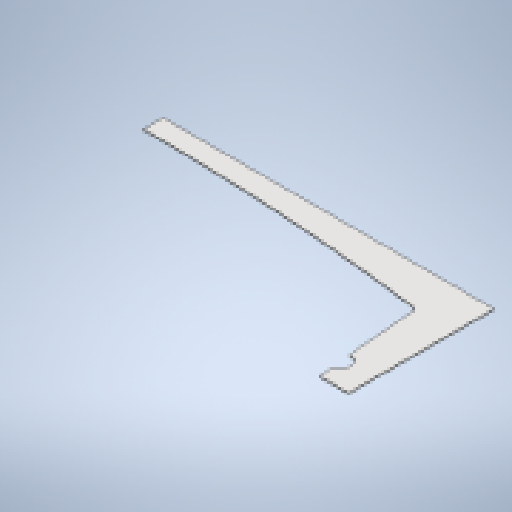
# Autodesk Inventor part: МОО 041 шпангоут спина 1
Saved by Autodesk Inventor 2024.2 (Build 282272000, 272)
## iProperties
Created: 2024-04-28
Part Number: МОО 041 шпангоут спина 1
Material: Generic
Document SubType Name: Sheet Metal
Designer: admin
Density: 1 g/cm^3
Sheet Metal Rule: Default_mm
Appearance: Default
Author: admin
Autodesk Inventor part; units mm, degrees
ref_plane "YZ Plane" through (0, 0, 0) normal (1, 0, 0) x (0, 1, 0)
ref_plane "XZ Plane" through (0, 0, 0) normal (0, 1, 0) x (-1, 0, 0)
ref_plane "XY Plane" through (0, 0, 0) normal (0, 0, 1) x (1, 0, 0)
sketch "Sketch1" plane through (0, 0, 0) normal (0, 0, 1) x (1, 0, 0)
  line L0 (-750, 0) -> (750, 0) construction
  line L1 (750, 0) -> (750, -2700) construction
  line L2 (750, -2700) -> (-750, -2700) construction
  line L3 (-750, -2700) -> (-750, 0) construction
  line L4 (800, 50) -> (-800, 50) construction
  line L5 (-800, 50) -> (-800, -2750) construction
  line L6 (-800, -2750) -> (800, -2750) construction
  line L7 (800, -2750) -> (800, 50) construction
  line L8 (-850, 100) -> (850, 100)
  line L9 (850, 100) -> (850, -2800) construction
  line L10 (850, -2800) -> (-850, -2800) construction
  line L11 (-850, -2800) -> (-850, 100) construction
  arc A0 (750, 0) -> (745.2706, 0.6314) centre (0, -5600) ccw construction
  line L12 (-750, -2100) -> (750, -2100) construction
  line L13 (114.1118, -2698.3696) -> (750, -2100) construction
  arc A1 (750, -2100) -> (770.156, -238.4205) centre (-10250, -1050) ccw construction
  line L14 (750, 0) -> (749.6018, -2.9735) construction
  arc A2 (750, -3.0268) -> (0, 47) centre (-0.2, -5603) ccw construction
  line L15 (750, 0) -> (747.0136, -0.2851) construction
  arc A3 (767.1641, -238.6409) -> (747.4657, -5.0326) centre (-10252.9895, -1050.2527) ccw construction
  arc A4 (750.4522, -4.7486) -> (745.2706, 0.6314) centre (744.4791, -5.3162) ccw
  arc A5 (747.4657, -5.0326) -> (744.8748, -2.3426) centre (744.4792, -5.3164) ccw construction
  line L16 (750, -2100) -> (752.9864, -2100.2851) construction
  arc A6 (752.9864, -2100.2851) -> (771.2831, -213.263) centre (-10246.9891, -1050.0292) ccw
  line L17 (750, -2100) -> (752.0559, -2102.1848) construction
  arc A7 (749.1768, -2100.7746) -> (750.1074, -2098.8746) centre (747.1209, -2098.5898) ccw construction
  line L18 (0, -2697) -> (110, -2697) construction
  line L19 (112.0559, -2696.1848) -> (690.4112, -2151.9536) construction
  arc A8 (110, -2700) -> (114.1118, -2698.3696) centre (110, -2694) ccw construction
  arc A9 (110, -2697) -> (112.0559, -2696.1848) centre (110, -2694) ccw construction
  line L20 (690.4112, -2151.9536) -> (692.4671, -2154.1384) construction
  line L21 (752.0559, -2102.1848) -> (676.3163, -2173.4556) construction
  line L22 (676.3163, -2173.4556) -> (674.2605, -2171.2708) construction
  arc A10 (747.4657, -5.0326) -> (747.0136, -0.2851) centre (-10252.9895, -1050.2527) ccw construction
  arc A11 (745.2706, 0.6314) -> (0, 50) centre (0, -5600) ccw
  arc A12 (750.4522, -4.7486) -> (750, 0) centre (-10250, -1050) ccw construction
  line L23 (770.156, -238.4205) -> (767.1641, -238.6409) construction
  line L24 (768.2917, -213.4901) -> (771.2831, -213.263) construction
  arc A13 (770.156, -238.4205) -> (750.4522, -4.7486) centre (-10250, -1050) ccw
  line L25 (0, 100) -> (0, 50)
  line L26 (0, -2700) -> (0, -2697) construction
  line L27 (0, 47) -> (0, 0) construction
  line L28 (0, 50) -> (0, 47) construction
  arc A14 (752.0559, -2102.1848) -> (752.9864, -2100.2851) centre (749.9998, -2099.9999) ccw construction
  circle A15 centre (768.2917, -213.4901) radius 25
  line L29 (850, -253.0064) -> (774.6194, -258.4205)
  arc A16 (800, 50) -> (0, 100) centre (0, -6325) ccw construction
  arc A17 (824.491, -254.8386) -> (800, 50) centre (-10587.7814, -1018.3062) ccw construction
  line L30 (824.491, -254.8386) -> (824.491, 100)
  point P0 (0, 0)
  point P1 (0, 0)
  point P2 (0, -2750)
  point P3 (766.3709, -188.564)
  point P4 (773.135, -238.0165)
  dimension "d6" = 1500
  dimension "d7" = 2700
  dimension "d8" = 2100
  dimension "d9" = 6
  dimension "d10" = 3
  dimension "d11" = 3
  dimension "d12" = 6
  dimension "d13" = 3
  dimension "d14" = 239.271
  dimension "d15" = 50
  dimension "d16" = 50
  dimension "d17" = 3
  dimension "d18" = 110
  dimension "d19" = 25
  dimension "d20" = 104
  dimension "d21" = 25
  dimension "d34" = 20
  dimension "d35" = 50
  measures "d6" distance of L3.end L1.start
  measures "d7" distance of L1.start L1.end
  measures "d8" distance between parallel lines of L12 L0
  measures "d9" radius of A4
  measures "d10" radius of A5
  measures "d11" radius of A7
  measures "d12" radius of A8
  measures "d13" radius of A9
  measures "d14" distance of L23.start L1.start
  measures "d15" distance between parallel lines of L4 L8
  measures "d16" distance between parallel lines of L0 L4
  measures "d17" distance of L28.start L27.start
  measures "d18" distance from line of L26 A8.centre
  measures "d19" distance of L22.end L20.end
  measures "d20" distance of L16.start L22.end
  measures "d21" distance of L23.start L24.start
  measures "d34" vertical distance of L23.start L29.end
  measures "d35" distance of L30.start L29.end
extrude "Plate1" add sketch "Sketch1" along normal blind 3 contours L8 L30 L29 A6 A15 A13 A4 A11 L25
equation "\"d6\" = d22"
equation "\"d7\" = d23"
equation "\"d8\" = d24"
equation "\"d9\" = d25"
equation "\"d10\" = d26"
equation "\"d11\" = d27"
equation "\"d12\" = d27 + d31"
equation "\"d13\" = d27"
equation "\"d14\" = d28"
equation "\"d17\" = d27"
equation "\"d18\" = 0.5 * d32"
equation "\"d19\" = d29"
equation "\"d20\" = d30"
equation "\"d21\" = d29"
equation "\"d35\" = d15"
equation "\"d5\" = Thickness"
equation "\"BendRadius\" = Thickness"
equation "\"BendReliefWidth\" = Thickness"
equation "\"BendReliefDepth\" = 0.5 * Thickness"
equation "\"CornerReliefSize\" = 4 * Thickness"
equation "\"MinimumRemnant\" = 2 * Thickness"
equation "\"TransitionRadius\" = BendRadius"
equation "\"JacobiRadiusSize\" = BendRadius"
equation "\"GapSize\" = Thickness"
equation "\"d25\" = d27 + d31"
equation "\"d26\" = d27"
equation "\"d31\" = d27"
equation "\"d22\" = 1500"
equation "\"d23\" = 2700"
equation "\"d24\" = 2100"
equation "\"d27\" = 3"
equation "\"d28\" = 239.271"
equation "\"d32\" = 220"
equation "\"d29\" = 25"
equation "\"d30\" = 104"
equation "\"Thickness\" = 3"
body "Solid1"
